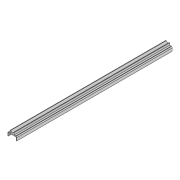
# Autodesk Inventor part: Base soporte tubos
Saved by Autodesk Inventor 2021 (Build 250183000, 183)
## iProperties
Created: 2021-04-30
Part Number: Base soporte tubos
Material: Generic
Document SubType Name: Modeling
Designer: Nelson
Density: 1 g/cm^3
Appearance: Default
Author: Nelson
Autodesk Inventor part; units mm, degrees
ref_plane "YZ Plane" through (0, 0, 0) normal (1, 0, 0) x (0, 1, 0)
ref_plane "XZ Plane" through (0, 0, 0) normal (0, 1, 0) x (-1, 0, 0)
ref_plane "XY Plane" through (0, 0, 0) normal (0, 0, 1) x (1, 0, 0)
sketch "Sketch1" plane through (0, 0, 0) normal (0, 0, 1) x (1, 0, 0)
  line L0 (-100, 0) -> (-100, 70)
  line L1 (-90, 80) -> (90, 80)
  line L2 (100, 70) -> (100, 0)
  arc A0 (-90, 80) -> (-100, 70) centre (-90, 70) ccw
  arc A1 (100, 70) -> (90, 80) centre (90, 70) ccw
  line L3 (-110, 0) -> (-110, 70)
  arc A2 (-90, 90) -> (-110, 70) centre (-90, 70) ccw
  arc A3 (110, 70) -> (90, 90) centre (90, 70) ccw
  line L4 (110, 70) -> (110, 0)
  line L5 (100, 0) -> (110, 0)
  line L6 (-100, 0) -> (-110, 0)
  line L7 (-90, 90) -> (-90, 100)
  line L8 (90, 90) -> (90, 100)
  line L9 (-50, 100) -> (-50, 152)
  line L10 (50, 100) -> (50, 152)
  line L11 (-38, 152) -> (0, 115)
  line L12 (0, 115) -> (38, 152)
  line L13 (-50, 152) -> (-38, 152)
  line L14 (38, 152) -> (50, 152)
  line L15 (-90, 100) -> (-50, 100)
  line L16 (50, 100) -> (90, 100)
  point P0 (0, 0)
  dimension "d0" = 100
  dimension "d1" = 100
  dimension "d2" = 80
  dimension "d4" = 10
  dimension "d5" = 10
  dimension "d24" = 10
  dimension "d25" = 50
  dimension "d26" = 50
  dimension "d31" = 12
  dimension "d32" = 12
  dimension "d33" = 50
  dimension "d37" = 15
  dimension "d38" = 20
  dimension "d39" = 20
  dimension "d40" = 52
  dimension "d41" = 52
  constraints: 34 end point, 8 point on circle, 6 perpendicular, 4 centre point, 4 tangent, 4 vertical, 2 horizontal, 1 equal radius, 1 other
  measures "d0" distance from line of point (0, 0) L0
  measures "d1" distance from line of L2 point (0, 0)
  measures "d2" distance from line of L1 point (0, 0)
  measures "d4" radius of A0
  measures "d5" distance between parallel lines of L0 L3
  measures "d24" distance of L7.start L7.end
  measures "d25" distance from line of L9 point (0, 0)
  measures "d26" distance from line of L10 point (0, 0)
  measures "d31" distance of L9.end L11.start
  measures "d32" distance of L12.end L10.end
  measures "d33" distance from line of L9 L11.end
  measures "d37" distance from line of L16 L11.end
  measures "d38" distance between parallel lines of L1 L15
  measures "d39" distance between parallel lines of L1 L16
  measures "d40" distance between parallel lines of L15 L13
  measures "d41" distance between parallel lines of L16 L14
extrude "Extrusion1" add sketch "Sketch1" against normal blind 3850
equation "\"d26\" = d25"
equation "\"d33\" = d25"
equation "\"d39\" = d38"
equation "\"d41\" = d40"
equation "\"d36\" = d34"
equation "\"d34\" = 75"
body "Solid1"
